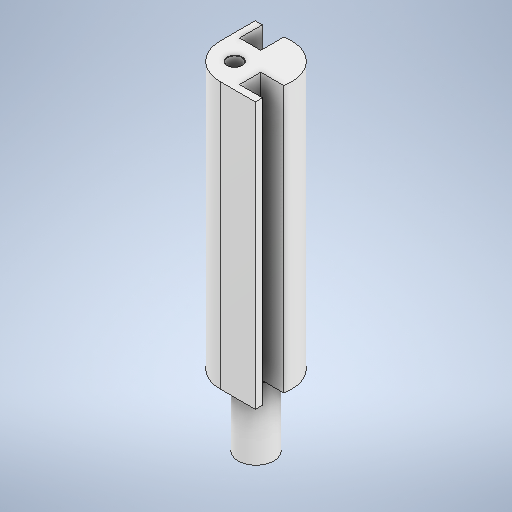
# Autodesk Inventor part: filar(5)
Saved by Autodesk Inventor 2025.2 (Build 292293000, 293)
## iProperties
Created: 2026-06-02
Part Number: filar(5)
Material: ABS Plastic
Document SubType Name: Modeling
Designer: ksawe
Density: 1.06 g/cm^3
Appearance: Smooth - White
Author: ksawe
Autodesk Inventor part; units mm, degrees
ref_plane "YZ Plane" through (0, 0, 0) normal (1, 0, 0) x (0, 1, 0)
ref_plane "XZ Plane" through (0, 0, 0) normal (0, 1, 0) x (-1, 0, 0)
ref_plane "XY Plane" through (0, 0, 0) normal (0, 0, 1) x (1, 0, 0)
sketch "Sketch1" plane through (0, 0, 0) normal (0, 1, 0) x (-1, 0, 0)
  circle A0 centre (0, 0) radius 10
  circle A1 centre (0, 0) radius 5
  line L0 (8, 0) -> (8, -6)
  line L1 (2, -4.5826) -> (2, -9.798)
  line L2 (10, 0) -> (5, 0)
  line L3 (7.0711, 7.0711) -> (-7.0711, -7.0711) construction
  line L4 (0, 8) -> (-6, 8)
  line L5 (-4.5826, 2) -> (-9.798, 2)
  line L6 (0, 10) -> (0, 5)
  line L7 (10, 0) -> (10, -9.798)
  line L8 (10, -9.798) -> (2, -9.798)
  line L9 (0, 10) -> (-9.798, 10)
  line L10 (-9.798, 10) -> (-9.798, 2)
  line L11 (-4.5826, 2) -> (0, 2)
  line L12 (0, 2) -> (0, 5)
  line L13 (5, 0) -> (2, 0)
  line L14 (2, 0) -> (2, -4.5826)
  line L15 (-6, 8) -> (-9.798, 8)
  line L16 (8, -6) -> (8, -9.798)
  line L17 (-3.345, 2) -> (-3.345, 9.4239)
  line L18 (2, -3.345) -> (9.4239, -3.345)
  point P0 (-9.798, 2)
  point P1 (8, -3.345)
  point P2 (-3.345, 8)
  point P3 (-9.798, 2)
  dimension "d0" = 20
  dimension "d1" = 10
  dimension "d10" = 6
  dimension "d11" = 2
  dimension "d12" = 45
  dimension "d15" = 3.3451
  constraints: 38 end point, 8 point on circle, 8 symmetric about line, 6 perpendicular, 6 point on line, 3 horizontal, 2 centre point, 2 coincident, 2 vertical, 1 horizontal alignment, 1 midpoint, 1 parallel, 1 tangent
  measures "d0" diameter of A0
  measures "d1" diameter of A1
  measures "d10" distance between parallel lines of L1 L0
  measures "d11" distance of L2.start L0.start
  measures "d12" angle of L2 L3
  measures "d15" distance between parallel lines of L6 L17
extrude "Extrusion1" add sketch "Sketch1" along normal blind 95 contours L2 A1 L6 A0 | L7 L8 L16 A0 | A0 L18 L0 L2 | L6 L4 L17 A0 | A0 L15 L10 L9 | A0 L0 L18 | L0 L18 A1 L2 | L17 L4 A0 | L6 A1 L17 L4 | L13 L14 A1 L11 L12 | A1 L18 L14 L13 | L12 L11 L17 A1 | A0 L5 A1 L1
extrude "Extrusion2" cut sketch "Sketch1" along normal blind 20 contours L2 A1 L6 A0 | L7 L8 L16 A0 | A0 L18 L0 L2 | L6 L4 L17 A0 | A0 L15 L10 L9 | A0 L0 L18 | L0 L18 A1 L2 | L17 L4 A0 | L6 A1 L17 L4 | A0 L1 A1 L18 L0 | L4 L17 A1 L5 A0 | A0 L10 L15 | A0 L5 A1 L1
extrude "Extrusion3" add sketch "Sketch1" along normal blind 20 contours A1 L18 L14 L13 | L12 L11 L17 A1 | A1 L14 L18 | L17 L11 A1
sketch "Sketch2" plane through (0, 95, 0) normal (0, 1, 0) x (1, 0, 0)
  line L0 (-10, 9.798) -> (-10, 0) projected
  line L1 (0, -10) -> (9.798, -10) projected
  point P0 (0, 0)
  point P1 (-3, -3)
  dimension "d16" = 7
  dimension "d24" = 7
  measures "d16" distance from line of L0 point (-3, -3)
  measures "d24" distance from line of L1 point (-3, -3)
hole "Hole1" at (-3, 95, 3) direction (0, -1, 0) diameter 4 depth 7 countersink diameter 4.2 countersink angle 90
sketch "Sketch3" plane through (0, 0, 0) normal (0, -1, 0) x (1, 0, 0)
  circle A0 centre (0, 0) radius 5 projected
  constraints: 1 coincident
hole "Hole2" at (0, 0, 0) direction (0, 1, 0) diameter 4 depth 7 countersink diameter 4.2 countersink angle 90
body "Solid1"
